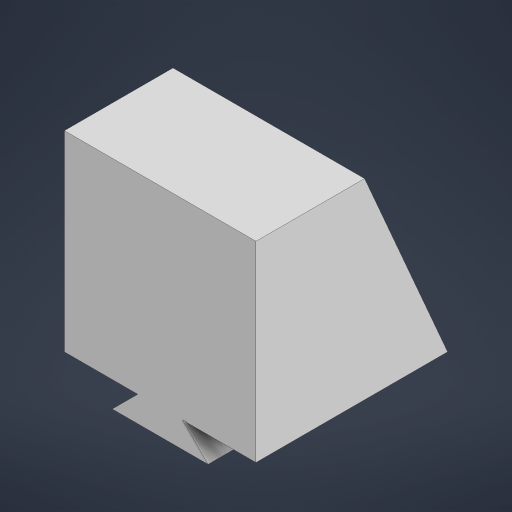
# Autodesk Inventor part: CarlaRescueRampeTeil2
Saved by Autodesk Inventor 2024 (Build 280153000, 153)
## iProperties
Created: 2024-01-16
Part Number: CarlaRescueRampeTeil2
Material: Generisch
Document SubType Name: Modeling
Designer: Robotik
Density: 1 g/cm^3
Appearance: Vorgabe
Author: Robotik
Autodesk Inventor part; units mm, degrees
ref_plane "YZ Plane" through (0, 0, 0) normal (1, 0, 0) x (0, 1, 0)
ref_plane "XZ Plane" through (0, 0, 0) normal (0, 1, 0) x (-1, 0, 0)
ref_plane "XY Plane" through (0, 0, 0) normal (0, 0, 1) x (1, 0, 0)
sketch "Skizze1" plane through (0, 0, 0) normal (1, 0, 0) x (0, 1, 0)
  line L0 (-8.5, -15) -> (8.5, -15)
  line L1 (8.5, -15) -> (8.5, 15)
  line L2 (8.5, 15) -> (-8.5, 15)
  line L3 (-8.5, 15) -> (-8.5, -15)
  line L4 (-8.5, -15) -> (8.5, 15) construction
  line L5 (8.5, -15) -> (-8.5, 15) construction
  line L6 (-8.5, -15) -> (21.5, -15)
  line L7 (21.5, -15) -> (8.5, 15)
  point P0 (0, 0)
  point P1 (8.5, -15)
  dimension "d0" = 30
  dimension "d1" = 17
  dimension "d3" = 30
  constraints: 16 end point, 2 midpoint, 2 parallel, 1 horizontal, 1 perpendicular, 1 point on line
  measures "d0" distance of L0.end L1.end
  measures "d1" distance of L1.end L2.end
  measures "d3" distance of L0.start L6.end
extrude "Extrusion1" add sketch "Skizze1" along normal blind 30
sketch "Skizze2" plane through (0, -8.5, -15) normal (0, 0, -1) x (-1, 0, 0)
  line L0 (0, 30) -> (-30, 30) construction
  line L1 (-15, 30) -> (-15, 0) construction
  line L2 (0, 0) -> (-30, 0) construction
  line L3 (0, 17) -> (0, 0) construction
  line L4 (0, 15) -> (-30, 15) construction
  circle A0 centre (-15, 15) radius 2.15
  point P0 (0, 8.5)
  dimension "d6" = 4.3
  constraints: 4 end point, 3 midpoint, 1 centre point, 1 horizontal, 1 point on line
  measures "d6" diameter of A0
extrude "Extrusion2" cut sketch "Skizze2" against normal blind 2
sketch "Skizze4" plane through (0, -8.5, -15) normal (0, -1, 0) x (1, 0, 0)
  line L0 (0, 30) -> (30, 30) construction
  line L1 (15, 30) -> (15, 0) construction
  line L2 (17.15, 0) -> (12.85, 0) construction
  line L3 (7.5, 4) -> (22.5, 4)
  line L4 (0, 0) -> (30, 0) projected
  line L5 (0, 30) -> (0, 0) projected
  line L6 (7.5, 4) -> (11.5, 0)
  line L7 (0, 0) -> (30, 0) projected
  line L8 (22.5, 4) -> (18.5, 0)
  line L9 (7.5, -4) -> (22.5, -4)
  line L10 (7.5, -4) -> (11.5, 0)
  line L11 (22.5, -4) -> (18.5, 0)
  point P0 (0, 15)
  dimension "d9" = 4
  dimension "d10" = 15
  dimension "d11" = 7.5
  dimension "d12" = 45
  constraints: 14 end point, 2 midpoint, 2 point on line, 2 symmetric about line, 1 horizontal, 1 vertical
  measures "d9" distance between parallel lines of L4 L3
  measures "d10" distance of L3.start L3.end
  measures "d11" distance from line of L5 L3.start
  measures "d12" angle of L4 L6
extrude "Extrusion3" add sketch "Skizze4" against normal blind 30 contours L4 L11 L9 L10
